# Autodesk Inventor part: 25-00000E_TEMPLATE_TOP
Saved by Autodesk Inventor 2025.3 (Build 293356000, 356)
## iProperties
Manager: Baum, R Chase
Company: DIS-TRAN STEEL, LLC
RuleStatus: InUse
Created: 2020-12-21
Document SubType Name: Sheet Metal
Mass: 63591.2 g
Surface Area: 17791 cm^2
Volume: 8100.8 cm^3
Density: 7.85 g/cm^3
Engr Approved By: Eng. Approved By
User Status: 1
Material: A572 GRADE 65
Sheet Metal Rule: DTS_PLATE_.375_(3/8)
Appearance: A572 GRADE 65 - APPEARANCE
Description: =<STEEL_DESIGNATION> <Thickness>x<BEARING_PLATE_DIA>
Sheet Metal Width: 48.750 in
Sheet Metal Length: 48.750 in
Sheet Metal Area: 2376.563 in^2
Part Number: 25-00000E_TEMPLATE_TOP
Flat Pattern Width: 123.825 cm
Flat Pattern Length: 123.825 cm
Flat Pattern Area: 15332.6 cm^2
Project: ONCOR TEMPLATE
Designer: I.C. NUTHING
Engineer: JSA
AfterDocOpen0: file://iLOGIC - ANY-ALL COMPONENTS\SET VISUAL STYLE
BeforeDocSave0: file://iLOGIC - ANY-ALL COMPONENTS\iProperty Update
BeforeDocSave1: file://iLOGIC - ANY-ALL COMPONENTS\Perform Weight Calculations
BeforeDocSave2: SEPARATE DIAMETER INTO FEET AND INCHES FOR BOM
STEEL_GRADE: A572 GRADE 65
REMARK (A): (WELD)
PRODUCT_DESIGNATION: PL
CUSTOMER: DTPS
ITEM_NUMBER: 01
JOB_NAME: Sloan Canyon
P.O._NUMBER: 12345
PART_NAME: FLANGE PLATE
PROJECT_LOCATION: SOMEWHERE, SOME TOWN, SOME STATE
DESCRIPTION: PL 3/8x
STEEL_DESIGNATION: PL
Thickness: 3/8
REMARKS: =<REMARK (A)><REMARK (B)><REMARK (C)>
JOB_NUMBER: 24-16975P
PLATE_THICKNESS: 0.375
SURFACE_SQ_FT: 15.521 ft^2
SHEET_METAL_THICKNESS: .1875_INCH
DATE_TIME_STAMP: 2505141436
PART_ORIGIN: F
COMPANY: DTSF
PLANT: MfgSys
ASSEMBLYSEQ: 6
PARENTASSEMBLYSEQ: 5
PRIORPEER: -1.0
BOMSEQUENCE: 600
BOMLEVEL: 3
QTYPER: 1
CHARACTER01: =<Revision Number>
NUMBER01: 0
NUMBER02: 0
NUMBER03: 0
NUMBER04: 0
NUMBER05: 0
NUMBER06: 0
NUMBER07: 0
NUMBER08: 0
NUMBER09: 0
NUMBER10: 0
NUMBER11: 0
NUMBER12: 0
NUMBER13: 0
NUMBER14: 1.0
NUMBER15: 0
CHECKBOX01: NO
CHECKBOX03: NO
CHEMINS_C: NO
CHEMOUT_C: NO
UVOUTSIDE_C: NO
NUMBER19: 0.0
DIRECT_BUY: NO
IT_PARTNUM: NO
IUM: lbs
MTLSEQ: 1465.0
VENDORNUM: 0
ORDERED: 0
MISCCHARGE: NO
ENABLEPURDIR: NO
DSPBUYIT: NO
SUBCONTRACT: NO
OPRSEQ: 10;
OPCODE: WELD;
VENDORID: MILLEN01
FINALOPR: NO
PIECEMARK: =<MarkPrefix><MARK><MarkSuffix>
MarkPrefix: 1
MarkSuffix: 1
STRUCT_NUM: =<MarkPrefix>
COMP_TYPE: PART
QTYSTR: 1
BOLT_CIRCLE_DIA: 42.0
JOBNUM: =<JOB_NUMBER>
PARTNUM: =<PIECEMARK>
NUMBER010: 0
NUMBER011: 0
NUMBER012: 0
NUMBER013: 0
MARK: a
STRUCTURE_DESCRIPTION: =<COMP_TYPE>-<Description>
PROJECT_NUMBER: 00
DETAIL_DESCRIPTION: ABC
CiPROP_LENGTH_FT: 3
CiPROP_LENGTH_IN: 9
FILE NAME: 25-00000E_TEMPLATE_TOP
SO_NUM: 20
CHEMTHANE_INSIDE_A: False
CHEMTHANE_OUTSIDE_A: False
HOLES_DRILLED_A: False
DEGLARE_A: False
UV_INSIDE_A: False
UV_OUTSIDE_A: False
BOM DESC: PL 3/8x
SURFACE SQ FT: 19.15 ft^2
BLACK WEIGHT: 141.0
WEIGHT AFTER GALV: 146.0
DocNumber: BASE_PL1.ipt
Folder: .\
VDS_Category: Engineering
NO_OF_BOLTS: 12
BOLT_CIRCLE: 41.5
MATERIAL: A572-65
Excel file path: C:\DTS_InventorWork\Designs\Engineering\Inventor Models\Excel Spreadsheets\XX_DESCRIPTION_OUTB_VWZ_PL_V2.0 - INVENTOR TEST.xlsm
BASEPLATE_R_EMBEDDED: BASE PLATE
BOLT_HOLE_DIA: 42.25
BOLT_SPACING_ANG: 15.0
DRAIN_HOLE_DIA: 25.0
GALVANIZED: YES
HOLE_SIZE: 2.75
HOLE_SPACING: 6.0
NO_SIDES: 12
NUM_BOLT_HOLES: 12
SHAFT_SHAPE: 12
WIDTH_IN: 48.75
WIDTH_FT: 4.0625
TEMPLATE_CENTER_HOLE_DIA: 25
TEMPLATE_DIA: 48 3/4
INPUT_TEMPLATE_DIAMETER: 48 3/4
TEMPLATE_BOT_GAP: 1.0
TEMPLATE_BOT_THK: 0.375
TEMPLATE_TOP_HOLE_SZ: 2.3125
TEMPLATE_TOP_THK: 0.5
THREAD_LEN: 12.0
VNOTCH: 0
TEMPLATE_RAD: 24 3/8
Author: Budden, Shawn A
Title: =<FILE NAME>-<Project>-<CUSTOMER>
Subject: MASTER ASSEMBLY
Keywords: FLANGE, PLATE
Revision Number: REV A
Autodesk Inventor part; units mm, degrees
ref_plane "UCSBasePlConstraintOrigin: YZ Plane" through (0, 0, 0) normal (0, 0, -1) x (0, 1, 0)
ref_plane "UCSBasePlConstraintOrigin: XZ Plane" through (0, 0, 0) normal (0, 1, 0) x (1, 0, 0)
ref_plane "BASE_PLATE_FACE" through (9.525, 0, 0) normal (1, 0, 0) x (0, 1, 0)
sketch "BASE_PLATE_SKETCH" plane through (9.525, 0, 0) normal (1, 0, 0) x (0, 0, -1)
  circle A0 centre (0, 0) radius 536.575 construction
  circle A1 centre (0, 0) radius 317.5
  line L0 (0, 536.575) -> (0, 536.575) construction
  circle A2 centre (0, 0) radius 619.125
  line L1 (0, 0) -> (-52.5935, -533.9912) construction
  line L2 (0, 0) -> (52.5935, -533.9912) construction
  line L3 (313.0592, 52.9167) -> (404.7136, 0)
  line L4 (404.7136, 0) -> (313.0592, -52.9167)
  line L5 (313.0592, -52.9167) -> (313.0592, 52.9167)
  line L6 (0, 0) -> (0, 536.575) construction
  line L7 (0, 0) -> (267.5578, 465.1081) construction
  point P0 (-619.125, 0)
  point P1 (619.125, 0)
  point P2 (0, 619.125)
  point P3 (0, -619.125)
  point P4 (0, 619.125)
  point P5 (619.125, 0)
  point P6 (0, -619.125)
  point P7 (-619.125, 0)
  point P8 (343.6107, 0)
  point P9 (313.0592, 0)
  point P10 (313.0592, -52.9167)
  dimension "GapSize" = 9.525
  dimension "SeamGap" = 0.0051
  dimension "Thickness" = 9.525
  dimension "BendRadius" = 9.525
  dimension "MinimumRemnant" = 19.05
  dimension "BendReliefDepth" = 4.7625
  dimension "BendReliefWidth" = 9.525
  dimension "CornerReliefSize" = 38.1
  dimension "JacobiRadiusSize" = 9.525
  dimension "TransitionRadius" = 9.525
  dimension "TEMPLATE_CENTER_HOLE_DIA" = 635
  dimension "NUMBER_OF_HOLES_IN_BOLT_PLATE" = 12
  dimension "BOLT_CIRCLE_DIA" = 1073.15
  dimension "TEMPLATE_DIA" = 1238.25
  dimension "PARENT_HOLE_ANG_L" = 5.625
  dimension "PARENT_HOLE_ANG_R" = 5.625
  dimension "NOTCH_LEG" = 105.8333
  dimension "d297" = 105.8333
  dimension "LEADER_PLACE_A_ANG" = 29.91
  constraints: 18 end point, 10 point on circle, 8 coincident, 2 centre point, 2 horizontal alignment, 2 vertical, 1 midpoint, 1 point on line, 10 other
  measures "BOLT_CIRCLE_DIA" diameter of A0
  measures "TEMPLATE_DIA" diameter of A2
  measures "PARENT_HOLE_ANG_L" angle of L1 L0
  measures "PARENT_HOLE_ANG_R" angle of L2 L0
  measures "NOTCH_LEG" distance of L3.start L3.end
  measures "d297" distance of L4.end L3.start
  measures "LEADER_PLACE_A_ANG" angle of L7 L6
extrude "BASE_PLATE_BODY" add sketch "BASE_PLATE_SKETCH" against normal up to surface (9.525 mm away) contours A1 L3 L4 | A2
ref_plane "SHAFT_MOUNTING_PLANE" through (9.525, 0, 0) normal (1, 0, 0) x (0, 1, 0)
hole "PARENT_HOLE" at (9.525, -533.9912, -52.5935) direction (-1, 0, 0) diameter 58.7375 depth 9.525 tip angle 118
pattern_circular "BOLT_HOLES" count 12 over 360 about axis through (-10, 0, 0) along (1, 0, 0) of "PARENT_HOLE"
ref_plane "DimPlaneRight" through (0, 0, -619.125) normal (0, 0, 1) x (1, 0, 0)
ref_plane "DimPlaneLeft" through (0, 0, 619.125) normal (0, 0, 1) x (1, 0, 0)
ref_plane "DimPlaneTop" through (0, 619.125, 0) normal (0, 1, 0) x (-1, 0, 0)
ref_plane "DimPlaneBtm" through (0, -619.125, 0) normal (0, 1, 0) x (-1, 0, 0)
ref_plane "PLPointBngPltCenterHoleDia" through (0, 0, 0) normal (0, -0.866, 0.5) x (1, 0, 0)
extrude "V NOTCH CUT" cut sketch "BASE_PLATE_SKETCH" against normal through all contours A1 L3 L4
equation "\"BOLT_CIRCLE_DIA\" = INPUT_BOLT_CIRCLE_DIAMETER"
equation "\"INPUT_TEMPLATE_DIAMETER\" = 1238.25"
equation "\"INPUT_BOLT_HOLE_SIZE\" = 58.7375"
equation "\"INPUT_BOLT_CIRCLE_DIAMETER\" = 1073.15"
equation "\"INPUT_PARENT_HOLE_ANG_OFF_90_270\" = 5.625deg"
equation "\"SHAFT_B_DIST_AK_BOTTOM\" = 933.5008"
equation "\"SHAFT_B_DIST_AF_BOTTOM\" = 901.7"
equation "\"SHAFT_B_Thickness\" = 7.9502"
equation "\"INPUT_CENTER_HOLE_DIAMETER\" = 635"
equation "\"LEADER_PLACE_A\" = 68.5deg"
equation "\"TEMPLATE_RAD\" = 619.125"
